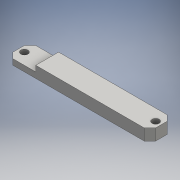
# Autodesk Inventor part: promo_arm1
Saved by Autodesk Inventor 2016 (Build 200138000, 138)
## iProperties
Created: 2016-05-11
Part Number: promo_arm1
Material: 一般
Document SubType Name: Modeling
Designer: 宏太
Density: 1 g/cm^3
Appearance: 既定
Mass: 0.906548 g
Surface Area: 9.2143 cm^2
Volume: 0.906548 cm^3
Author: 宏太
Autodesk Inventor part; units mm, degrees
ref_plane "YZ Plane" through (0, 0, 0) normal (1, 0, 0) x (0, 1, 0)
ref_plane "XZ Plane" through (0, 0, 0) normal (0, 1, 0) x (-1, 0, 0)
ref_plane "XY Plane" through (0, 0, 0) normal (0, 0, 1) x (1, 0, 0)
sketch "スケッチ1" plane through (0, 0, 0) normal (0, 1, 0) x (-1, 0, 0)
  line L0 (-25, -2) -> (25, -2)
  line L1 (25, -2) -> (25, 2)
  line L2 (25, 2) -> (-25, 2)
  line L3 (-25, 2) -> (-25, -2)
  line L4 (-25, -2) -> (25, 2) construction
  line L5 (25, -2) -> (-25, 2) construction
  point P0 (0, 0)
  dimension "d0" = 50
  dimension "d1" = 4
  constraints: 12 end point, 2 midpoint, 2 parallel, 1 horizontal, 1 perpendicular
  measures "d0" distance of L2.end L1.end
  measures "d1" distance of L1.end L0.end
extrude "押し出し1" add sketch "スケッチ1" along normal mid plane 8
sketch "スケッチ2" plane through (0, 0, 0) normal (0, 0, 1) x (1, 0, 0)
  circle A0 centre (-23, 0) radius 1.25
  line L0 (-25, -4) -> (-25, 4) projected
  circle A1 centre (23, 0) radius 1.25
  line L1 (25, -4) -> (25, 4) projected
  point P0 (0, 0)
  dimension "d4" = 2.5
  dimension "d5" = 2
  dimension "d14" = 2.5
  dimension "d15" = 2
  constraints: 2 centre point
  measures "d4" diameter of A0
  measures "d5" distance from line of L0 A0.centre
  measures "d14" diameter of A1
  measures "d15" distance from line of L1 A1.centre
extrude "押し出し2" cut sketch "スケッチ2" along normal mid plane 5 contours A0
chamfer "面取り1" distance 2 angle 45 1 edges at (-25, 4, 0)
chamfer "面取り2" distance 2 angle 45 1 edges at (-25, -4, 0)
sketch "スケッチ3" plane through (0, 0, 0) normal (0, 0, 1) x (1, 0, 0)
  circle A0 centre (23, 0) radius 1.25
  line L0 (25, -4) -> (25, 4) projected
  point P0 (0, 0)
  dimension "d16" = 2.5
  dimension "d17" = 2
  constraints: 1 centre point
  measures "d16" diameter of A0
  measures "d17" distance from line of L0 A0.centre
extrude "押し出し3" cut sketch "スケッチ3" along normal mid plane 5
chamfer "面取り3" distance 2 angle 45 1 edges at (25, 4, 0)
chamfer "面取り4" distance 2 angle 45 1 edges at (25, -4, 0)
sketch "スケッチ4" plane through (0, -4, 0) normal (0, -1, 0) x (1, 0, 0)
  line L0 (-25, -2) -> (-25, 2) projected
  line L1 (-25, 0) -> (-15, 0)
  line L2 (-15, 0) -> (-15, 2)
  line L3 (-15, 2) -> (-25, 2)
  line L4 (-25, 2) -> (-25, 0)
  point P0 (0, 0)
  dimension "d26" = 10
  constraints: 8 end point, 2 parallel, 1 horizontal, 1 midpoint, 1 perpendicular
  measures "d26" distance of L3.end L2.end
extrude "押し出し4" cut sketch "スケッチ4" against normal blind 10
